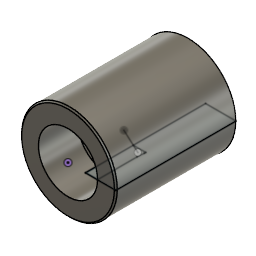
CASING WITH SINGLE SIDE BORE (Autodesk Fusion 360 design; units mm, degrees)
Autodesk Fusion 360 part; units mm, degrees
sketch "Sketch1" plane through (0, 0, 0) normal (0, 1, 0) x (1, 0, 0)
  line L0 (25.4635, 63.881) -> (9.3726, 63.881)
  line L1 (9.3726, 63.881) -> (9.3726, 0)
  line L2 (9.3726, 0) -> (25.4635, 0)
  line L3 (25.4635, 0) -> (25.4635, 63.881)
  line L4 (15.7353, 0) -> (15.7353, 21.0056)
  line L5 (15.7353, 21.0056) -> (15.9893, 24.638)
  line L6 (15.9893, 24.638) -> (15.9893, 25.4)
  line L7 (15.9893, 25.4) -> (9.3726, 25.4)
  line L8 (0, 29.7705) -> (13.8983, 23.2896)
  dimension "d1" = 9.3726
  dimension "d2" = 25.4635
  dimension "d3" = 63.881
  dimension "d6" = 15.7353
  dimension "d7" = 0.762
  dimension "d8" = 4
  dimension "d9" = 25.4
  dimension "d10" = 0.254
  dimension "d11" = 65
  constraint horizontal L0
  constraint vertical L1
  constraint horizontal L2
  constraint vertical L3
  constraint horizontal origin L1.end
  constraint coincident L2 L4.start
  constraint perpendicular L2 L4
  constraint perpendicular L2 L6
  constraint coincident L1 L7.end
  constraint perpendicular L1 L7
  constraint vertical origin L8.start
  constraint coincident L7.end L8
  measures "d1" distance of origin L1
  measures "d2" distance of origin L2.end
  measures "d3" distance of L0.start L2.end
  measures "d6" distance of origin L4
  measures "d7" distance of L5.end L6.end
  measures "d8" angle of L4 L5
  measures "d9" distance of L2 L7
  measures "d10" distance of L4 L6
  measures "d11" angle of L3 L8
revolve "Revolve1" add sketch "Sketch1" angle 360 about axis through (0, 0, 1.75) along (0, 0, 1) contours L0 L1 L2 L3 L4 L5 L6 L7
chamfer "Chamfer1" distance 0.762 angle 45 1 edges at (-23.7403, -9.208, 0)
equation "d1 = ( 0.738 / 2 ) * 1 in"
equation "d2 = 2.005 in / 2"
equation "d3 = 2.5 in + 0.015 in"
equation "d6 = ( 1.239 / 2 ) * 1 in"
equation "d11 = ( 130 / 2 ) * 1 deg"
